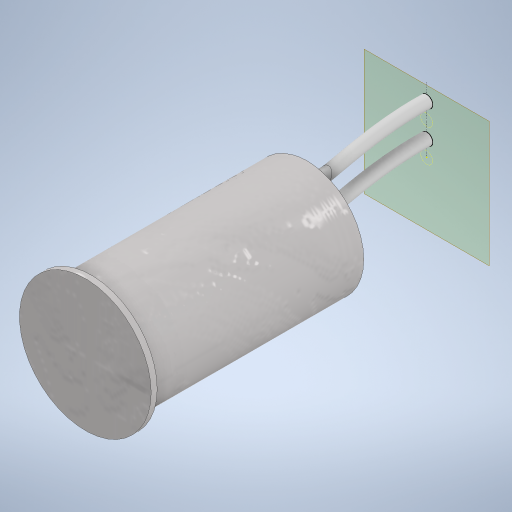
# Autodesk Inventor part: capteur_tirette_fixe
Saved by Autodesk Inventor 2024.2 (Build 282272000, 272)
## iProperties
Created: 2023-11-11
Part Number: capteur_tirette_fixe
Material: Generic
Document SubType Name: Modeling
Designer: adrie
Density: 1 g/cm^3
Appearance: Default
Author: adrie
Autodesk Inventor part; units mm, degrees
ref_plane "YZ Plane" through (0, 0, 0) normal (1, 0, 0) x (0, 1, 0)
ref_plane "XZ Plane" through (0, 0, 0) normal (0, 1, 0) x (-1, 0, 0)
ref_plane "XY Plane" through (0, 0, 0) normal (0, 0, 1) x (1, 0, 0)
sketch "Sketch1" plane through (0, 0, 0) normal (0, 0, 1) x (1, 0, 0)
  circle A0 centre (0, 0) radius 4.75
  dimension "d0" = 9.5
  constraints: 1 centre point, 1 coincident
  measures "d0" diameter of A0
extrude "Extrusion1" add sketch "Sketch1" along normal blind 18
sketch "Sketch2" plane through (0, 0, 18) normal (0, 0, 1) x (1, 0, 0)
  circle A0 centre (0, 0) radius 5.5
  dimension "d4" = 11
  constraints: 1 centre point, 1 coincident
  measures "d4" diameter of A0
extrude "Extrusion2" add sketch "Sketch2" along normal blind 0.5
sketch "Sketch3" plane through (0, 0, 0) normal (0, 0, -1) x (-1, 0, 0)
  circle A0 centre (0, 0) radius 0.5
  circle A1 centre (0, 2.7139) radius 0.5
  dimension "d7" = 1
  constraints: 2 centre point, 1 coincident, 1 equal radius
  measures "d7" diameter of A1
ref_plane "Work Plane2" through (0, 0, -10) normal (0, 0, -1) x (-1, 0, 0)
sketch "Sketch4" plane through (0, 0, -10) normal (0, 0, -1) x (-1, 0, 0)
  circle A0 centre (0, 0) radius 0.5 construction
  circle A1 centre (0, 2.7139) radius 0.5 construction
  line L0 (0, 2.7139) -> (0, 0) construction
  line L1 (0, 2.7139) -> (0, 5.4278) construction
  circle A2 centre (0, 1.357) radius 0.5
  circle A3 centre (0, 4.0709) radius 0.5
  constraints: 4 end point, 2 centre point, 2 equal radius, 2 midpoint, 2 vertical, 1 collinear
sketch "Sketch5" plane through (0, 0, 0) normal (1, 0, 0) x (0, 1, 0)
  line L0 (2.7139, 0) -> (3.0133, -2.5875) construction
  line L1 (3.0133, -2.5875) -> (4.1868, -5.4698) construction
  line L2 (4.1868, -5.4698) -> (4.0709, -10) construction
  spline S0 degree 3 poles (2.7139, 0) (3.0133, -2.5875) (4.1868, -5.4698) (4.0709, -10) knots 1 1 1 1 2 2 2 2
  spline S1 degree 4 poles (0.018, -0.3119) (0.1484, -1.4472) (0.3995, -2.5637) (0.9656, -4.9307) (1.3253, -7.343) (1.3902, -8.6392) (1.3578, -9.9306) knots 0 0 0 0 0 0.469122 0.469122 1 1 1 1 1
  point P0 (0, 0)
  point P1 (1.357, -10)
  point P2 (0, 0)
  constraints: 6 other
sweep "Sweep1" add profiles "Sketch3" path "Sketch5" keep normal constant yes path curves S0
fillet "Fillet1" radius 1.5 2 edges at (0.5, 2.7139, 0) (0.5, 0, 0)
body "Solid1"
